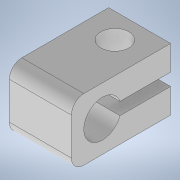
# Autodesk Inventor part: BT15_Klemme
Saved by Autodesk Inventor 2022 (Build 260153000, 153)
## iProperties
Created: 2022-01-06
Part Number: BT15_Klemme
Material: Generic
Document SubType Name: Modeling
Designer: Rayen
Density: 1 g/cm^3
Appearance: Default
Author: Rayen
Autodesk Inventor part; units mm, degrees
ref_plane "YZ Plane" through (0, 0, 0) normal (1, 0, 0) x (0, 1, 0)
ref_plane "XZ Plane" through (0, 0, 0) normal (0, 1, 0) x (-1, 0, 0)
ref_plane "XY Plane" through (0, 0, 0) normal (0, 0, 1) x (1, 0, 0)
sketch "Sketch1" plane through (0, 0, 0) normal (0, 0, 1) x (1, 0, 0)
  line L0 (344.9937, 353.3773) -> (-355.0063, 353.3773)
  line L1 (-455.0063, 253.3773) -> (-455.0063, -46.6227)
  line L2 (-355.0063, -146.6227) -> (344.9937, -146.6227)
  line L3 (344.9937, -146.6227) -> (344.9937, 53.3773)
  line L4 (344.9937, 153.3773) -> (344.9937, 353.3773)
  arc A0 (-63.585, 153.3773) -> (-63.585, 53.3773) centre (-205.0063, 103.3773) ccw
  line L5 (344.9937, 153.3773) -> (-63.585, 153.3773)
  line L6 (344.9937, 53.3773) -> (-63.585, 53.3773)
  arc A1 (-355.0063, 353.3773) -> (-455.0063, 253.3773) centre (-355.0063, 253.3773) ccw
  arc A2 (-455.0063, -46.6227) -> (-355.0063, -146.6227) centre (-355.0063, -46.6227) ccw
  point P0 (0, 0)
  point P1 (-455.0063, 353.3773)
  point P2 (-455.0063, -146.6227)
  dimension "d0" = 800
  dimension "d1" = 500
  dimension "d8" = 250
  dimension "d9" = 300
  dimension "d10" = 100
  dimension "d11" = 100
  dimension "d12" = 200
  dimension "d13" = 200
  constraints: 14 end point, 6 point on circle, 4 perpendicular, 4 point on line, 4 tangent, 3 centre point, 2 horizontal, 1 equal radius, 1 parallel
  measures "d0" distance of L0.start point (-455.006, 353.377)
  measures "d1" distance of point (-455.006, 353.377) point (-455.006, -146.623)
  measures "d8" distance from line of L1 A0.centre
  measures "d9" diameter of A0
  measures "d10" radius of A1
  measures "d11" distance between parallel lines of L6 L5
  measures "d12" distance of L4.start L0.start
  measures "d13" distance of L2.end L3.end
extrude "Extrusion1" add sketch "Sketch1" along normal blind 500
sketch "Sketch2" plane through (-355.0063, 353.3773, 0) normal (0, 1, 0) x (1, 0, 0)
  circle A0 centre (500, -250) radius 112.7771
  line L0 (700, -500) -> (0, -500) projected
  line L1 (700, 0) -> (700, -500) projected
  point P0 (355.0063, 0)
  dimension "d16" = 250
  dimension "d17" = 200
  constraints: 1 centre point
  measures "d16" distance from line of L0 A0.centre
  measures "d17" distance from line of L1 A0.centre
extrude "Extrusion2" cut sketch "Sketch2" against normal blind 700
body "Solid1"
